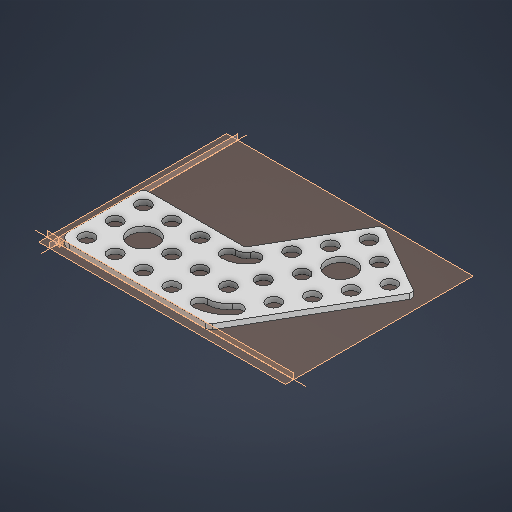
# Autodesk Inventor part: bend plate
Saved by Autodesk Inventor 2026.1 (Build 301233020, 233B)
## iProperties
Created: 2025-10-18
Part Number: bend plate
Material: Generic
Document SubType Name: Modeling
Designer: User
Density: 1 g/cm^3
Appearance: Default
Author: User
Autodesk Inventor part; units mm, degrees
sketch "Sketch1" plane through (0, 0, 0) normal (0, 1, 0) x (-1, 0, 0)
  line L0 (-3.0271, 0) -> (-41.6123, 0)
  line L1 (-42.4778, 0) -> (0, 0) construction
  line L2 (0, -3.0271) -> (0, -22.5589)
  line L3 (0, 0) -> (-4, 0)
  circle A0 centre (-4, -4) radius 2
  circle A1 centre (-4, -12) radius 2
  circle A2 centre (-4, -20) radius 2
  circle A3 centre (-12, -12) radius 4
  circle A4 centre (-12, -20) radius 2
  circle A5 centre (-20, -20) radius 2
  circle A6 centre (-20, -12) radius 2
  circle A7 centre (-12, -4) radius 2
  circle A8 centre (-20, -4) radius 2
  circle A9 centre (-28, -4) radius 2
  circle A10 centre (-28, -12) radius 2
  arc A11 (-28.0533, -21.9993) -> (-28, -18) centre (-28, -20) ccw
  arc A12 (-36, -6) -> (-36.2624, -2.0173) centre (-36, -4) ccw
  circle A13 centre (-36, -12) radius 2
  circle A14 centre (-36.4295, -29.4856) radius 2
  circle A15 centre (-40.4295, -36.4138) radius 2
  arc A16 (-34.1615, -21.5574) -> (-30.6714, -23.5108) centre (-32.4295, -22.5574) ccw
  arc A17 (-28, -22) -> (-30.6974, -23.5574) centre (-28.0667, -24.9993) ccw
  arc A18 (-28, -18) -> (-34.1615, -21.5574) centre (-28.0667, -24.9993) ccw
  circle A19 centre (-44.4295, -43.342) radius 2
  circle A20 centre (-51.3577, -39.342) radius 2
  circle A21 centre (-47.3577, -32.4138) radius 4
  circle A22 centre (-43.3577, -25.4856) radius 2
  circle A23 centre (-39.3577, -18.5574) radius 2
  arc A24 (-43.9199, -6.2146) -> (-40.6974, -8.5482) centre (-42.4295, -7.5482) ccw
  arc A25 (-36, -2) -> (-44.1615, -6.5482) centre (-35.4324, -12.6153) ccw
  arc A26 (-36, -6) -> (-40.6974, -8.5482) centre (-35.8127, -11.9491) ccw
  line L4 (0, -3.0271) -> (0, -22.4904)
  line L5 (-1.5, -23.9904) -> (-27.8558, -23.9904)
  line L6 (-42.2835, -47.5041) -> (-29.1552, -24.741)
  arc A27 (-27.8558, -23.9904) -> (-29.1552, -24.741) centre (-27.8558, -25.4904) ccw
  arc A28 (-44.2827, -48.0814) -> (-42.2835, -47.5041) centre (-43.5829, -46.7547) ccw
  arc A29 (-1.5, -23.9904) -> (0, -22.4904) centre (-1.5, -22.4904) ccw
  arc A30 (0, -3.0271) -> (-3.0271, 0) centre (-3.0271, -3.0271) ccw
  arc A31 (-41.6123, 0) -> (-42.9109, -0.7493) centre (-41.6123, -1.5) ccw
  arc A32 (-64.169, -37.5251) -> (-64.1463, -37.6038) centre (-64.1198, -37.5536) ccw
  circle A33 centre (-58.2817, -35.3348) radius 2
  circle A34 centre (-54.2817, -28.4066) radius 2
  circle A35 centre (-50.2817, -21.4784) radius 2
  line L7 (-42.9109, -0.7493) -> (-0.4781, -0.7493) construction
  line L8 (-44.2827, -48.0814) -> (-62.8833, -37.3424)
  line L9 (-63.2493, -35.9764) -> (-42.9109, -0.7493)
  arc A36 (-63.2493, -35.9764) -> (-62.8833, -37.3424) centre (-62.3833, -36.4764) ccw
  circle A37 centre (-46.2817, -14.5502) radius 2
  point P0 (0, 0)
  point P1 (0, -23.9904)
  constraints: 38 centre point, 38 point on circle, 20 end point, 10 tangent, 7 point on line, 4 horizontal, 1 concentric, 1 equal radius, 1 vertical
extrude "Extrusion1" add sketch "Sketch1" along normal blind 1.5
body "Solid1"
